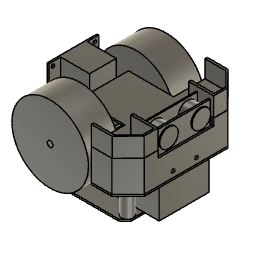
SUMO ROBOT (Autodesk Fusion 360 design; units mm, degrees)
Autodesk Fusion 360 part; units mm, degrees
note: some values were not read from the file. Chosen so that the rebuilt part matches the saved one: which face or edge a step refers to.
(part 1 of 2)
sketch "Sketch1" plane through (0, 0, 0) normal (0, 0, 1) x (1, 0, 0)
  line L0 (0, 0) -> (100, 0)
  line L1 (100, 0) -> (100, 100)
  line L2 (100, 100) -> (0, 100)
  line L3 (0, 100) -> (0, 0)
  constraint horizontal L0
  constraint vertical L1
  constraint horizontal L2
  constraint vertical L3
  constraint coincident L0.start L3.end
sketch "Sketch2" plane through (0, 0, 0) normal (0, 0, 1) x (1, 0, 0)
  line L0 (125, 0) -> (147, 0)
  line L1 (147, 0) -> (147, 19)
  line L2 (147, 19) -> (125, 19)
  line L3 (125, 19) -> (125, 0)
  dimension "d1" = 22
  dimension "d2" = 19
  constraint horizontal L0
  constraint vertical L1
  constraint horizontal L2
  constraint vertical L3
  measures "d1" distance of L0.start L0.end
  measures "d2" distance of L0.start L2.end
extrude "Extrude1" add sketch "Sketch2" against normal blind 64 makes body 1
sketch "Sketch3" plane through (0, 0, -64) normal (0, 0, -1) x (1, 0, 0)
  line L0 (125, 0) -> (125, -19)
  line L1 (125, -19) -> (147, -19)
  line L2 (147, -19) -> (147, 0)
  line L3 (147, 0) -> (125, 0)
extrude "Extrude2" cut sketch "Sketch3" against normal blind 27 bodies 1
extrude "Extrude3" add 1 faces at (132.3333, 12.6667, 0) along direction (0, 0, 1) blind 27 separate body on bodies 1 makes body 2
move_face "OffsetFaces1" offset -2.5 4 faces at (147, 6.3333, 18) (132.3333, 0, 9) (125, 12.6667, 18) (139.6667, 19, 9) on bodies 2
fillet "Fillet1" radius 5 2 edges at (147, 9.5, -37) (125, 9.5, -37) on bodies 1
sketch "Sketch4" plane through (0, 0, 0) normal (0, -1, 0) x (1, 0, 0)
  arc A0 (125, -32) -> (130, -37) centre (130, -32) ccw
  line L0 (130, -37) -> (142, -37)
  arc A1 (142, -37) -> (147, -32) centre (142, -32) ccw
  line L1 (147, -32) -> (147, 0)
  line L2 (147, 0) -> (125, 0)
  line L3 (125, 0) -> (125, -32)
  line L4 (130, -37) -> (130, -7)
  line L5 (125, -7.4905) -> (126, -7.4905)
  circle A2 centre (128, -7) radius 2
  circle A3 centre (144, -7) radius 2
  dimension "d12" = 4
  constraint coincident A0.end L0.start
  constraint perpendicular L0 L4
  constraint coincident L3 L5.start
  constraint perpendicular L3 L5
  measures "d12" diameter of A2
extrude "Extrude4" cut sketch "Sketch4" against normal blind 71 contours A2 | A3 bodies 1
sketch "Sketch5" plane through (0, 0, 0) normal (0, -1, 0) x (1, 0, 0)
  circle A0 centre (128, -7) radius 2
  circle A1 centre (144, -7) radius 2
  arc A2 (125, -32) -> (130, -37) centre (130, -32) ccw
  line L0 (130, -37) -> (142, -37)
  arc A3 (142, -37) -> (147, -32) centre (142, -32) ccw
  line L1 (147, -32) -> (147, 0)
  line L2 (147, 0) -> (125, 0)
  line L3 (125, 0) -> (125, -32)
  line L4 (136, -37) -> (136, -28)
  line L5 (136, -28) -> (136, -25.5)
  circle A4 centre (136, -25.5) radius 2.5
  dimension "d15" = 2.5
  constraint midpoint L0 L4.start
  constraint perpendicular L0 L4
  constraint parallel L4 L5
  constraint coincident L5.end A4.centre
  constraint coincident L4.end A4
  measures "d15" distance of L4.end L5.end
extrude "Extrude5" add sketch "Sketch5" along normal blind 9 and the other way blind 28 contours A4 bodies 1
sketch "Sketch6" plane through (0, -9, 0) normal (0, -1, 0) x (1, 0, 0)
  circle A0 centre (136, -25.5) radius 2.5
  circle A1 centre (136, -25.5) radius 33
  dimension "d20" = 66
  constraint concentric A0 A1
  measures "d20" diameter of A1
extrude "Extrude6" add sketch "Sketch6" along normal blind 26 separate body makes body 3
move_body "Move1" bodies 3 to x (1, 0, 0) y (0, 1, 0) z (0, 0, 1) at (0, 6, 0)
move_body "Move2" bodies 2 3 1 to x (0, 0, -1) y (0, 1, 0) z (1, 0, 0) at (135, 0, 121)
copy_body "CopyPasteBodies1" bodies 1 3 2 makes body 4 makes body 5 makes body 6
move_body "Move3" bodies 4 5 6 to x (1, 0, 0) y (0, -1, 0) z (0, 0, -1) at (0, 72, -30)
move_body "Move4" bodies 5 4 6 to x (1, 0, 0) y (0, 1, 0) z (0, 0, 1) at (-80, 0, 4)
move_body "Move5" bodies 3 1 2 to x (1, 0, 0) y (0, 1, 0) z (0, 0, 1) at (-80, 15, 4)
sketch "Sketch7" plane through (0, 0, 0) normal (0, 0, 1) x (1, 0, 0)
sketch "Sketch8" plane through (0, 0, 0) normal (0, 0, 1) x (1, 0, 0)
  line L0 (0, 72) -> (66, 72)
  line L1 (66, 72) -> (66, 15)
  line L2 (66, 15) -> (0, 15)
  line L3 (0, 15) -> (0, 72)
  line L4 (100, 100) -> (66, 100)
  line L5 (66, 100) -> (66, 0)
  line L6 (66, 0) -> (100, 0)
  line L7 (100, 0) -> (100, 100)
  constraint horizontal L0
  constraint vertical L1
  constraint horizontal L2
  constraint vertical L3
  constraint horizontal L4
  constraint vertical L5
  constraint horizontal L6
  constraint vertical L7
extrude "Extrude7" add sketch "Sketch8" along normal blind 2.5 separate body makes body 7
extrude "Extrude8" add 1 faces at (88.6667, 100, 1.6667) along direction (0, 1, 0) blind 1 on bodies 7 bodies 7
extrude "Extrude9" add 1 faces at (77.3333, 0, 1.6667) along direction (0, -1, 0) blind 14 on bodies 7 bodies 7
sketch "Sketch9" plane through (0, 53, 0) normal (0, -1, 0) x (1, 0, 0)
  circle A0 centre (29.5, -11) radius 2.5
  circle A1 centre (48, -19) radius 2
  circle A2 centre (48, -3) radius 2
  arc A3 (18, -17) -> (23, -22) centre (23, -17) ccw
  line L0 (23, -22) -> (55, -22)
  line L1 (55, -22) -> (55, 0)
  line L2 (55, 0) -> (23, 0)
  arc A4 (23, 0) -> (18, -5) centre (23, -5) ccw
  line L3 (18, -5) -> (18, -17)
  circle A5 centre (48, -19) radius 2
  circle A6 centre (48, -3) radius 2
  constraint concentric A1 A5
  constraint concentric A2 A6
sketch "Sketch10" plane through (0, 0, 0) normal (0, 0, -1) x (1, 0, 0)
  line L0 (66, 14) -> (66, -15)
  line L1 (66, -15) -> (0, -15)
  line L2 (0, -15) -> (0, -72)
  line L3 (0, -72) -> (66, -72)
  line L4 (66, -72) -> (66, -101)
  line L5 (66, -101) -> (100, -101)
  line L6 (100, -101) -> (100, 14)
  line L7 (100, 14) -> (66, 14)
  line L8 (42, -53) -> (54, -53)
  line L9 (54, -53) -> (54, -34)
  line L10 (54, -34) -> (42, -34)
  line L11 (42, -34) -> (42, -53)
  line L12 (42, -47) -> (54, -47)
  line L13 (54, -47) -> (54, -40)
  line L14 (54, -40) -> (42, -40)
  line L15 (42, -40) -> (42, -47)
  constraint horizontal L8
  constraint vertical L9
  constraint horizontal L10
  constraint vertical L11
  constraint horizontal L12
  constraint vertical L13
  constraint horizontal L14
  constraint vertical L15
  constraint coincident L9 L13.end
  constraint coincident L11 L12.start
extrude "Extrude10" add sketch "Sketch10" along normal blind 22 separate body contours L8 L9 L11 L12 | L9 L10 L11 L14 makes body 8 at (46, 47, -7.3333) makes body 9 at (50, 34, -7.3333)
extrude "Extrude11" cut sketch "Sketch9" along normal blind 40 contours A1 A5 | A2 A6 bodies 8 9
sketch "Sketch11" plane through (0, 0, 0) normal (0, 0, -1) x (1, 0, 0)
  line L0 (66, 14) -> (66, -15)
  line L1 (66, -15) -> (0, -15)
  line L2 (0, -15) -> (0, -72)
  line L3 (0, -72) -> (66, -72)
  line L4 (66, -72) -> (66, -101)
  line L5 (66, -101) -> (100, -101)
  line L6 (100, -101) -> (100, 14)
  line L7 (100, 14) -> (66, 14)
  circle A0 centre (95, -50) radius 1.5
  circle A1 centre (95, -43) radius 2
  dimension "d33" = 3
  measures "d33" diameter of A0
extrude "Extrude12" cut sketch "Sketch11" against normal blind 5 contours A0 | A1 bodies 7
sketch "Sketch12" plane through (0, 0, 0) normal (1, 0, 0) x (0, 1, 0)
  line L0 (-55, 0) -> (-100, 0)
  line L1 (-100, 0) -> (-100, 20)
  line L2 (-100, 20) -> (-55, 20)
  line L3 (-55, 20) -> (-55, 0)
  circle A0 centre (-65, 10) radius 8
  circle A1 centre (-90, 10) radius 8
  dimension "d36" = 45
  dimension "d37" = 20
  dimension "d38" = 16
  dimension "d39" = 16
  constraint horizontal L0
  constraint vertical L1
  constraint horizontal L2
  constraint vertical L3
  measures "d36" distance of L0.start L0.end
  measures "d37" distance of L0.start L2.end
  measures "d38" diameter of A0
  measures "d39" diameter of A1
extrude "Extrude13" add sketch "Sketch12" along normal blind 1 separate body makes body 10
extrude "Extrude14" add sketch "Sketch12" along normal blind 13 contours A0 | A1 bodies 10
move_body "Move6" bodies 10 to x (1, 0, 0) y (0, 1, 0) z (0, 0, 1) at (86, 121, -35)
sketch "Sketch13" plane through (87, 0, 0) normal (1, 0, 0) x (0, 1, 0)
  circle A0 centre (56, -25) radius 8
  circle A1 centre (31, -25) radius 8
  line L0 (66, -15) -> (21, -15)
  line L1 (21, -15) -> (21, -35)
  line L2 (21, -35) -> (66, -35)
  line L3 (66, -35) -> (66, -15)
  line L4 (22, -34) -> (65, -34)
  line L5 (65, -34) -> (65, 0)
  line L6 (65, 0) -> (22, 0)
  line L7 (22, 0) -> (22, -34)
  circle A2 centre (56, -25) radius 8
  circle A3 centre (31, -25) radius 8
  constraint horizontal L4
  constraint vertical L5
  constraint horizontal L6
  constraint vertical L7
  constraint concentric A0 A2
  constraint concentric A1 A3
extrude "Extrude15" add sketch "Sketch13" along normal blind 3 contours L0 L4 L5 L7 | L0 L5 L6 L7 bodies 7
chamfer "Chamfer1" distance 2 angle 45 4 edges at (90, 43.5, 0) (88.5, 65, 0) (88.5, 22, 0) (87, 43.5, 0) on bodies 7
chamfer "Chamfer2" distance 10 angle 45 2 edges at (100, -14, 1.25) (100, 101, 1.25) on bodies 7
sketch "Sketch14" plane through (0, 0, 0) normal (0, 0, -1) x (1, 0, 0)
  line L0 (90, -101) -> (100, -91)
  line L1 (100, -91) -> (100, 4)
  line L2 (100, 4) -> (90, 14)
  line L3 (90, 14) -> (66, 14)
  line L4 (66, 14) -> (66, -15)
  line L5 (66, -15) -> (0, -15)
  line L6 (0, -15) -> (0, -72)
  line L7 (0, -72) -> (66, -72)
  line L8 (66, -72) -> (66, -101)
  line L9 (66, -101) -> (90, -101)
  circle A0 centre (95, -43) radius 2
  circle A1 centre (95, -50) radius 1.5
  line L10 (85, -20) -> (92, -20)
  line L11 (92, -20) -> (92, -67)
  line L12 (92, -67) -> (85, -67)
  line L13 (85, -67) -> (85, -20)
  circle A2 centre (90, 9) radius 2
  circle A3 centre (93, 5) radius 1.5
  circle A4 centre (90, -95) radius 2
  circle A5 centre (93, -90) radius 1.5
  dimension "d48" = 3
  dimension "d49" = 3
  measures "d48" diameter of A3
  measures "d49" diameter of A5
extrude "Extrude16" cut sketch "Sketch14" against normal blind 5 contours A2 | A3 | A4 | A5 bodies 7
sketch "Sketch15" plane through (0, 0, 0) normal (1, 0, 0) x (0, 1, 0)
  line L0 (-60, 0) -> (-103, 0)
  line L1 (-103, 0) -> (-103, 43)
  line L2 (-103, 43) -> (-60, 43)
  line L3 (-60, 43) -> (-60, 0)
  line L4 (-81.5, 4.9861) -> (-70, 4.9861)
  line L5 (-70, 4.9861) -> (-70, 0)
  line L6 (-70, 0) -> (-81.5, 0)
  line L7 (-81.5, 0) -> (-81.5, 4.9861)
  line L8 (-81.5, 4.9861) -> (-93, 4.9861)
  line L9 (-93, 4.9861) -> (-93, 0)
  line L10 (-93, 0) -> (-81.5, 0)
  line L11 (-81.5, 0) -> (-81.5, 4.9861)
  line L12 (-70, 0) -> (-93, 0)
  line L13 (-93, 0) -> (-93, 16)
  line L14 (-93, 16) -> (-70, 16)
  line L15 (-70, 16) -> (-70, 0)
  dimension "d52" = 43
  dimension "d53" = 43
  constraint horizontal L0
  constraint vertical L1
  constraint horizontal L2
  constraint vertical L3
  constraint horizontal L4
  constraint vertical L5
  constraint horizontal L6
  constraint vertical L7
  constraint coincident L0 L5.end
  constraint horizontal L8
  constraint vertical L9
  constraint horizontal L10
  constraint vertical L11
  constraint coincident L0 L9.end
  constraint horizontal L12
  constraint vertical L13
  constraint horizontal L14
  constraint vertical L15
  measures "d52" distance of L0.start L0.end
  measures "d53" distance of L0.start L2.end
extrude "Extrude17" add sketch "Sketch15" along normal blind 1.5 separate body makes body 11
extrude "Extrude18" add sketch "Sketch15" against normal blind 25 contours L0 L4 L5 L6 L7 L11 L12 L15 | L0 L7 L8 L9 L10 L11 L12 L13 | L4 L8 L13 L14 L15 bodies 11
sketch "Sketch16" plane through (1.5, 0, 0) normal (1, 0, 0) x (0, 1, 0)
  line L0 (-103, 0) -> (-60, 0)
  line L1 (-60, 0) -> (-60, 43)
  line L2 (-60, 43) -> (-103, 43)
  line L3 (-103, 43) -> (-103, 0)
  line L4 (-60, 0) -> (-62, 0)
  line L5 (-60, 0) -> (-60, 2)
  line L6 (-60, 2) -> (-103, 2)
  line L7 (-62, 0) -> (-62, 43)
  circle A0 centre (-63.5, 3.5) radius 1.5
  line L8 (-101, 0) -> (-101, 43)
  line L9 (-62, 41) -> (-101, 41)
  circle A1 centre (-99.5, 3.5) radius 1.5
  circle A2 centre (-99.5, 39.5) radius 1.5
  circle A3 centre (-63.5, 39.5) radius 1.5
  constraint coincident L0.end L1.start
  constraint coincident L0 L4.end
  constraint perpendicular L1 L4
  constraint coincident L1 L5.end
  constraint coincident L3 L6.end
  constraint perpendicular L3 L6
  constraint coincident L2 L7.end
  constraint perpendicular L2 L7
  constraint tangent L6 A0
  constraint coincident L0 L8.start
  constraint coincident L2 L8.end
  constraint perpendicular L2 L8
  constraint coincident L7 L9.start
  constraint coincident L8 L9.end
  constraint perpendicular L8 L9
  constraint tangent L8 A1
  constraint tangent L8 A2
  constraint tangent L7 A3
extrude "Extrude19" cut sketch "Sketch16" against normal blind 10 contours A1 | A0 | A2 | A3 bodies 11
extrude "Extrude20" add 1 faces at (0, -85.3333, 31.2328) along direction (-1, 0, 0) blind 10 on bodies 11 bodies 11
move_body "Move7" bodies 11 to x (0, 0, -1) y (0, 1, 0) z (1, 0, 0) at (3, 125, -35)
move_body "Move8" bodies 11 to x (1, 0, 0) y (0, 1, 0) z (0, 0, 1) at (-2.5, 0, 0)
sketch "Sketch17" plane through (0, 0, -36.5) normal (0, 0, -1) x (1, 0, 0)
  circle A0 centre (4, -25.5) radius 1.5
  circle A1 centre (40, -25.5) radius 1.5
  circle A2 centre (4, -61.5) radius 1.5
  circle A3 centre (40, -61.5) radius 1.5
  line L0 (0.5, -22) -> (0.5, -65)
  line L1 (0.5, -65) -> (43.5, -65)
  line L2 (43.5, -65) -> (43.5, -22)
  line L3 (43.5, -22) -> (0.5, -22)
  circle A4 centre (4, -61.5) radius 1.5
  circle A5 centre (4, -25.5) radius 1.5
  constraint concentric A2 A4
  constraint concentric A0 A5
sketch "Sketch18" plane through (0, 0, -36.5) normal (0, 0, -1) x (1, 0, 0)
  circle A0 centre (4, -61.5) radius 3.5
  circle A1 centre (4, -25.5) radius 3.5
extrude "Extrude21" add sketch "Sketch18" against normal blind 35 separate body makes body 12 at (7.4826, 61.8485, -13.1667) makes body 13 at (7.4826, 25.8485, -13.1667)
extrude "Extrude22" cut sketch "Sketch17" against normal blind 55 contours A0 A5 | A2 A4 bodies 7 12 13
move_body "Move9" bodies 13 to x (1, 0, 0) y (0, 1, 0) z (0, 0, 1) at (0, 0, 4)
move_body "Move10" bodies 12 to x (1, 0, 0) y (0, 1, 0) z (0, 0, 1) at (0, 0, 4)
extrude "Extrude23" cut 2 faces at (3.2029, 28.2109, -32.5) (3.2029, 64.2109, -32.5) along direction (0, 0, 1) blind 10 on bodies 12 13 bodies 12 13
extrude "Extrude24" add 2 faces at (3.2029, 28.2109, -22.5) (3.2029, 64.2109, -22.5) along direction (0, 0, -1) blind 2.5 on bodies 12 13 bodies 13 12
sketch "Sketch19" plane through (0, 0, -22) normal (0, 0, -1) x (1, 0, 0)
  line L0 (42, -53) -> (54, -53)
  line L1 (54, -53) -> (54, -47)
  line L2 (54, -47) -> (42, -47)
  line L3 (42, -47) -> (42, -53)
  line L4 (42, -47) -> (54, -47)
  line L5 (54, -47) -> (54, -40)
  line L6 (54, -40) -> (42, -40)
  line L7 (42, -40) -> (42, -47)
  constraint horizontal L4
  constraint vertical L5
  constraint horizontal L6
  constraint vertical L7
  constraint coincident L2.end L3.start
extrude "Extrude25" cut sketch "Sketch19" against normal blind 37 contours L2 L4 L5 L6 L7 bodies 7
sketch "Sketch20" plane through (0, 0, 0) normal (0, 0, -1) x (1, 0, 0)
  line L0 (54, -47) -> (42, -47)
  line L1 (42, -47) -> (42, -40)
  line L2 (42, -40) -> (54, -40)
  line L3 (54, -40) -> (54, -47)
  circle A0 centre (4, -61.5) radius 1.5
  circle A1 centre (4, -25.5) radius 1.5
  circle A2 centre (93, 5) radius 1.5
  circle A3 centre (90, -95) radius 2
  circle A4 centre (90, 9) radius 2
  circle A5 centre (93, -90) radius 1.5
  line L4 (90, -101) -> (100, -91)
  line L5 (100, -91) -> (100, 4)
  line L6 (100, 4) -> (90, 14)
  line L7 (90, 14) -> (66, 14)
  line L8 (66, 14) -> (66, -15)
  line L9 (66, -15) -> (0, -15)
  line L10 (0, -15) -> (0, -72)
  line L11 (0, -72) -> (66, -72)
  line L12 (66, -72) -> (66, -101)
  line L13 (66, -101) -> (90, -101)
  circle A6 centre (95, -43) radius 2
  circle A7 centre (95, -50) radius 1.5
  line L14 (85, -20) -> (92, -20)
  line L15 (92, -20) -> (92, -67)
  line L16 (92, -67) -> (85, -67)
  line L17 (85, -67) -> (85, -20)
  circle A8 centre (75.2156, -86.5) radius 5
  circle A9 centre (75.2156, -0.5) radius 5
  dimension "d72" = 10
  dimension "d73" = 10
  measures "d72" diameter of A8
  measures "d73" diameter of A9
extrude "Extrude26" add sketch "Sketch20" along normal blind 40 contours A8 | A9 bodies 7
extrude "Extrude27" add 2 faces at (3.2029, 28.2109, -25) (3.2029, 64.2109, -25) along direction (0, 0, -1) blind 10 on bodies 12 13 bodies 13 12
sketch "Sketch21" plane through (0, 0, -40) normal (0, 0, -1) x (1, 0, 0)
  circle A0 centre (75.2156, -86.5) radius 5
  circle A1 centre (75.2156, -86.5) radius 1.5
  dimension "d78" = 3
  constraint concentric A0 A1
  measures "d78" diameter of A1
sketch "Sketch22" plane through (0, 0, -40) normal (0, 0, -1) x (1, 0, 0)
  circle A0 centre (75.2156, -0.5) radius 5
  circle A1 centre (75.2156, -0.5) radius 1.5
  dimension "d79" = 3
  constraint concentric A0 A1
  measures "d79" diameter of A1
extrude "Extrude28" cut sketch "Sketch22" sketch "Sketch21" against normal blind 72 contours A1 of sketch 2 contours A1 bodies 7
sketch "Sketch23" plane through (0, 0, -40) normal (0, 0, -1) x (1, 0, 0)
  circle A0 centre (75.2156, -86.5) radius 1.5
  circle A1 centre (75.2156, -86.5) radius 5
  line L0 (65, -101) -> (65, -72)
  line L1 (65, -72) -> (0, -72)
  line L2 (0, -72) -> (0, -15)
  line L3 (0, -15) -> (66, -15)
  line L4 (66, -15) -> (65, -15)
  line L5 (65, -15) -> (65, 14)
  line L6 (65, 14) -> (90, 14)
  line L7 (90, 14) -> (100, 4)
  line L8 (100, 4) -> (100, -91)
  line L9 (100, -91) -> (90, -101)
  line L10 (90, -101) -> (65, -101)
  constraint vertical L0
  constraint perpendicular L0 L1
  constraint perpendicular L1 L2
  constraint perpendicular L2 L3
  constraint coincident L3 L4.end
  constraint perpendicular L3 L5
  constraint perpendicular L5 L6
  constraint perpendicular L6 L8
  constraint perpendicular L7 L9
  constraint perpendicular L0 L10
extrude "Extrude29" add sketch "Sketch23" along normal blind 2.5 contours A1 | L0 L1 L2 L3 L5 L6 L7 L8 L9 L10 bodies 7
extrude "Extrude30" cut sketch "Sketch22" along normal blind 4 contours A1 bodies 7
sketch "Sketch24" plane through (0, 0, 0) normal (0, 0, 1) x (1, 0, 0)
  line L0 (-50, 0) -> (-115, 0)
  line L1 (-115, 0) -> (-115, 55)
  line L2 (-115, 55) -> (-50, 55)
  line L3 (-50, 55) -> (-50, 0)
  dimension "d86" = 65
  dimension "d87" = 55
  constraint horizontal L0
  constraint vertical L1
  constraint horizontal L2
  constraint vertical L3
  measures "d86" distance of L0.start L0.end
  measures "d87" distance of L0.start L2.end
sketch "Sketch25" plane through (0, 0, 0) normal (0, 0, 1) x (1, 0, 0)
extrude "Extrude31" add sketch "Sketch24" against normal blind 20 separate body makes body 14
chamfer "Chamfer3" distance 5 angle 45 4 edges at (-82.5, 0, -20) (-82.5, 55, -20) (-82.5, 0, 0) (-82.5, 55, 0) on bodies 14
move_body "Move11" bodies 14 to x (1, 0, 0) y (0, 1, 0) z (0, 0, 1) at (115, 17.5, -45)
sketch "Sketch26" plane through (0, 0, 0) normal (0, 1, 0) x (1, 0, 0)
  line L0 (-50, 0) -> (-117, 0)
  line L1 (-117, 0) -> (-117, -54)
  line L2 (-117, -54) -> (-50, -54)
  line L3 (-50, -54) -> (-50, 0)
  dimension "d91" = 67
  dimension "d92" = 54
  constraint horizontal L0
  constraint vertical L1
  constraint horizontal L2
  constraint vertical L3
  measures "d91" distance of L0.start L0.end
  measures "d92" distance of L0.start L2.end
extrude "Extrude32" add sketch "Sketch26" along normal blind 10 separate body makes body 15
move_body "Move12" bodies 15 to x (1, 0, 0) y (0, 0, 1) z (0, -1, 0) at (120, 72, -75)
sketch "Sketch27" plane through (0, 0, -75) normal (0, 0, -1) x (1, 0, 0)
  line L0 (70, -72) -> (70, -18)
  line L1 (70, -18) -> (3, -18)
  line L2 (3, -18) -> (3, -72)
  line L3 (3, -72) -> (70, -72)
  line L4 (3, -64.7927) -> (70, -64.7927)
  line L5 (70, -64.7927) -> (70, -25)
  line L6 (70, -25) -> (3, -25)
  line L7 (3, -25) -> (3, -64.7927)
  constraint horizontal L4
  constraint vertical L5
  constraint horizontal L6
  constraint vertical L7
  constraint coincident L0 L5.end
  constraint coincident L2 L4.start
extrude "Extrude33" cut sketch "Sketch27" against normal blind 5 contours L0 L2 L4 L5 L6 L7 bodies 15
move_body "Move13" bodies 14 15 to x (1, 0, 0) y (0, 1, 0) z (0, 0, 1) at (0, 0, 3)
sketch "Sketch28" plane through (100, 0, 0) normal (1, 0, 0) x (0, 1, 0)
  line L0 (91, -40) -> (-4, -40)
  line L1 (-4, -40) -> (-4, -42.5)
  line L2 (-4, -42.5) -> (91, -42.5)
  line L3 (91, -42.5) -> (91, -40)
  line L4 (-15.0228, -40) -> (107, -40)
  line L5 (107, -40) -> (107, -39.8)
  line L6 (107, -39.8) -> (-15.0228, -39.8)
  line L7 (-15.0228, -39.8) -> (-15.0228, -40)
  dimension "d97" = 0.2
  constraint horizontal L4
  constraint vertical L5
  constraint horizontal L6
  constraint vertical L7
  measures "d97" distance of L4.start L6.end
extrude "Extrude34" cut sketch "Sketch28" against normal blind 113 contours L0 L4 L5 L6 L7 bodies 7 makes body 16 at (17.3556, 42.3333, 2.5)
move_face "OffsetFaces2" offset -0.3 2 faces at (88, 63.9602, -25.7965) (89, 35.6699, -18.5045) on bodies 16
sketch "Sketch29" plane through (0, 53, 0) normal (0, 1, 0) x (-1, 0, 0)
  circle A0 centre (-48, -19) radius 2
  circle A1 centre (-48, -3) radius 2
  line L0 (-42, 0) -> (-54, 0)
  line L1 (-54, 0) -> (-54, -22)
  line L2 (-54, -22) -> (-42, -22)
  line L3 (-42, -22) -> (-42, 0)
  line L4 (-42, -22) -> (-42, 0)
  line L5 (-35, 0) -> (-42, -22)
  line L6 (-54, -22) -> (-54, 0)
  line L7 (-60, 0) -> (-54, -22)
  line L8 (-54, 0) -> (-60, 0)
  line L9 (-35, 0) -> (-42, 0)
  constraint coincident L2.end L3.start
  constraint coincident L0.start L3.end
  constraint coincident L1.end L2.start
  constraint coincident L0.end L1.start
  constraint perpendicular L6 L8
  constraint perpendicular L4 L9
extrude "Extrude35" add sketch "Sketch29" against normal blind 19 contours L3 L4 L5 L9 | L1 L6 L7 L8 bodies 8 9 16
sketch "Sketch30" plane through (0, 0, -22) normal (0, 0, -1) x (1, 0, 0)
  line L0 (42, -53) -> (54, -53)
  line L1 (54, -53) -> (54, -47)
  line L2 (54, -47) -> (42, -47)
  line L3 (42, -47) -> (42, -53)
  line L4 (65, -40) -> (30, -40)
  line L5 (30, -40) -> (30, -47)
  line L6 (30, -47) -> (65, -47)
  line L7 (65, -47) -> (65, -40)
  constraint horizontal L4
  constraint vertical L5
  constraint horizontal L6
  constraint vertical L7
extrude "Extrude36" cut sketch "Sketch30" against normal blind 34 contours L2 L4 L5 L6 L7 bodies 8
sketch "Sketch31" plane through (0, 0, 2.5) normal (0, 0, 1) x (-1, 0, 0)
  line L0 (-65, -40) -> (-30, -40)
  line L1 (-30, -40) -> (-30, -47)
  line L2 (-30, -47) -> (-65, -47)
  line L3 (-65, -47) -> (-65, -40)
  circle A0 centre (-75.2156, -0.5) radius 1.5
  circle A1 centre (-75.2156, -86.5) radius 1.5
  circle A2 centre (-4, -61.5) radius 1.5
  circle A3 centre (-4, -25.5) radius 1.5
  circle A4 centre (-93, 5) radius 1.5
  circle A5 centre (-90, -95) radius 2
  circle A6 centre (-90, 9) radius 2
  circle A7 centre (-93, -90) radius 1.5
  line L4 (-100, -91) -> (-90, -101)
  line L5 (-90, -101) -> (-66, -101)
  line L6 (-66, -101) -> (-66, -72)
  line L7 (-66, -72) -> (0, -72)
  line L8 (0, -72) -> (0, -15)
  line L9 (0, -15) -> (-66, -15)
  line L10 (-66, -15) -> (-66, 14)
  line L11 (-66, 14) -> (-90, 14)
  line L12 (-90, 14) -> (-100, 4)
  line L13 (-100, 4) -> (-100, -91)
  circle A8 centre (-95, -50) radius 1.5
  circle A9 centre (-95, -43) radius 2
  line L14 (-90, -55) -> (-80, -55)
  line L15 (-80, -55) -> (-80, -31)
  line L16 (-80, -31) -> (-90, -31)
  line L17 (-90, -31) -> (-90, -55)
  line L18 (-90, -55) -> (-80, -55)
  line L19 (-80, -55) -> (-80, -52)
  line L20 (-80, -52) -> (-90, -52)
  line L21 (-90, -52) -> (-90, -55)
  line L22 (-90, -31) -> (-80, -31)
  line L23 (-80, -31) -> (-80, -34)
  line L24 (-80, -34) -> (-90, -34)
  line L25 (-90, -34) -> (-90, -31)
  constraint horizontal L14
  constraint vertical L15
  constraint horizontal L16
  constraint vertical L17
  constraint horizontal L18
  constraint vertical L19
  constraint horizontal L20
  constraint vertical L21
  constraint coincident L15 L19.end
  constraint horizontal L22
  constraint vertical L23
  constraint horizontal L24
  constraint vertical L25
  constraint coincident L15 L23.end
extrude "Extrude37" add sketch "Sketch31" along normal blind 17 separate body contours L14 L15 L17 L18 L19 L20 L21 | L15 L16 L17 L22 L23 L24 L25 makes body 17 at (83.3333, 52, 8.1667) makes body 18 at (83.3333, 31, 8.1667)
sketch "Sketch32" plane through (0, 31, 0) normal (0, -1, 0) x (1, 0, 0)
  line L0 (80, 2.5) -> (90, 2.5)
  line L1 (90, 2.5) -> (90, 19.5)
  line L2 (90, 19.5) -> (80, 19.5)
  line L3 (80, 19.5) -> (80, 2.5)
  circle A0 centre (85, 15) radius 1.5
  dimension "d107" = 3
  measures "d107" diameter of A0
extrude "Extrude38" cut sketch "Sketch32" against normal blind 49 contours A0 bodies 17 18
chamfer "Chamfer4" distance 2 angle 45 4 edges at (80, 53.5, 19.5) (90, 53.5, 19.5) (90, 32.5, 19.5) (80, 32.5, 19.5) on bodies 17 18
sketch "Sketch33" plane through (0, 55, 0) normal (0, 1, 0) x (-1, 0, 0)
  line L0 (-88, 19.5) -> (-90, 17.5)
  line L1 (-90, 17.5) -> (-90, 2.5)
  line L2 (-90, 2.5) -> (-80, 2.5)
  line L3 (-80, 2.5) -> (-80, 17.5)
  line L4 (-80, 17.5) -> (-82, 19.5)
  line L5 (-82, 19.5) -> (-88, 19.5)
  circle A0 centre (-85, 15) radius 1.5
sketch "Sketch34" plane through (0, 0, 0) normal (1, 0, 0) x (0, 1, 0)
  line L0 (-50, -20) -> (-62, -20)
  line L1 (-62, -20) -> (-62, -3)
  line L2 (-62, -3) -> (-50, -3)
  line L3 (-50, -3) -> (-50, -20)
  line L4 (-56, -20) -> (-50, -13)
  line L5 (-56, -3) -> (-50, -10)
  line L6 (-56, -20) -> (-62, -13)
  line L7 (-62, -10) -> (-56, -3)
  line L8 (-56, -20) -> (-57.5, -20)
  line L9 (-57.5, -20) -> (-57.5, -3)
  line L10 (-57.5, -3) -> (-56, -3)
  line L11 (-56, -3) -> (-56, -20)
  line L12 (-56, -20) -> (-54.5, -20)
  line L13 (-54.5, -20) -> (-54.5, -3)
  line L14 (-54.5, -3) -> (-56, -3)
  line L15 (-56, -3) -> (-56, -20)
  dimension "d111" = 1.5
  dimension "d112" = 1.5
  constraint horizontal L0
  constraint vertical L1
  constraint horizontal L2
  constraint vertical L3
  constraint midpoint L0 L4.start
  constraint coincident L3 L4.end
  constraint midpoint L2 L5.start
  constraint coincident L3 L5.end
  constraint coincident L1 L6.end
  constraint parallel L5 L6
  constraint parallel L4 L7
  constraint horizontal L8
  constraint vertical L9
  constraint horizontal L10
  constraint vertical L11
  constraint horizontal L12
  constraint vertical L13
  constraint horizontal L14
  constraint vertical L15
  measures "d111" distance of L4.start L8.end
  measures "d112" distance of L4.start L12.end
revolve "Revolve1" add sketch "Sketch34" angle 360 about axis through (0, -56, -3) along (0, 0, -1) separate body contours L3 L4 L5 L13 makes body 19
move_body "Move14" bodies 19 to x (1, 0, 0) y (0, 0, -1) z (0, 1, 0) at (85, 56.25, -40.95)
move_body "Move15" bodies 19 to x (1, 0, 0) y (0, 1, 0) z (0, 0, 1) at (0, -1.5, 0)
sketch "Sketch35" plane through (0, -14, 0) normal (0, -1, 0) x (1, 0, 0)
  circle A0 centre (29.5, -11) radius 2.5
  circle A1 centre (29.5, -11) radius 33
sketch "Sketch36" plane through (0, 0, 2.5) normal (0, 0, 1) x (-1, 0, 0)
  line L0 (-65, -40) -> (-30, -40)
  line L1 (-30, -40) -> (-30, -47)
  line L2 (-30, -47) -> (-65, -47)
  line L3 (-65, -47) -> (-65, -40)
  circle A0 centre (-75.2156, -0.5) radius 1.5
  circle A1 centre (-75.2156, -86.5) radius 1.5
  circle A2 centre (-4, -61.5) radius 1.5
  circle A3 centre (-4, -25.5) radius 1.5
  circle A4 centre (-93, 5) radius 1.5
  circle A5 centre (-90, -95) radius 2
  circle A6 centre (-90, 9) radius 2
  circle A7 centre (-93, -90) radius 1.5
  line L4 (-100, -91) -> (-90, -101)
  line L5 (-90, -101) -> (-66, -101)
  line L6 (-66, -101) -> (-66, -72)
  line L7 (-66, -72) -> (0, -72)
  line L8 (0, -72) -> (0, -15)
  line L9 (0, -15) -> (-66, -15)
  line L10 (-66, -15) -> (-66, 14)
  line L11 (-66, 14) -> (-90, 14)
  line L12 (-90, 14) -> (-100, 4)
  line L13 (-100, 4) -> (-100, -91)
  circle A8 centre (-95, -50) radius 1.5
  circle A9 centre (-95, -43) radius 2
  line L14 (-66, -101) -> (-66, -102.5)
  line L15 (-66, -102.5) -> (-90, -102.5)
  line L16 (-90, -102.5) -> (-101.5, -91)
  line L17 (-101.5, -91) -> (-101.5, 4)
  line L18 (-101.5, 4) -> (-90, 15.5)
  line L19 (-90, 15.5) -> (-66, 15.5)
  line L20 (-66, 15.5) -> (-66, 14)
  constraint coincident L5.end L6.start
  constraint perpendicular L5 L14
  constraint perpendicular L6 L15
  constraint perpendicular L15 L17
  constraint parallel L12 L18
  constraint perpendicular L17 L19
  constraint coincident L10.end L11.start
  constraint perpendicular L11 L20
extrude "Extrude39" add sketch "Sketch36" against normal blind 15 separate body contours L4 L5 L11 L12 L13 L14 L15 L16 L17 L18 L19 L20 makes body 20
sketch "Sketch37" plane through (0, 102.5, 0) normal (0, 1, 0) x (-1, 0, 0)
  line L0 (-66, 2.5) -> (-90, 2.5)
  line L1 (-90, 2.5) -> (-90, -12.5)
  line L2 (-90, -12.5) -> (-66, -12.5)
  line L3 (-66, -12.5) -> (-66, 2.5)
  line L4 (-101.5, 2.5) -> (-120, 20)
  line L5 (-120, 20) -> (-118, 20)
  line L6 (-118, 20) -> (-100, 2.5)
  line L7 (-100, 2.5) -> (-101.5, 2.5)
  constraint horizontal L5
  constraint parallel L5 L7
extrude "Extrude40" add sketch "Sketch37" against normal blind 106.5 contours L4 L5 L6 L7 bodies 20
extrude "Extrude41" cut 1 faces at (113.1667, 102.5, 14.1667) along direction (0, -1, 0) blind 11.5 on bodies 20 bodies 20
sketch "Sketch38" plane through (0, 102.5, 0) normal (0, 1, 0) x (-1, 0, 0)
  line L0 (-66, 2.5) -> (-90, 2.5)
  line L1 (-90, 2.5) -> (-90, -12.5)
  line L2 (-90, -12.5) -> (-66, -12.5)
  line L3 (-66, -12.5) -> (-66, 2.5)
  line L4 (-90, 2.5) -> (-108.5, 20)
  line L5 (-108.5, 20) -> (-106.5, 20)
  line L6 (-106.5, 20) -> (-88.5, 2.5)
  constraint coincident L0.end L1.start
  constraint perpendicular L1 L5
  constraint coincident L0 L6.end
loft "Loft1" add profiles "Sketch38" section 1 face at (113.1667, 91, 14.1667) section 2 contours L0 L4 L5 L6 on bodies 20 bodies 20
sketch "Sketch39" plane through (0, -15.5, 0) normal (0, -1, 0) x (1, 0, 0)
  line L0 (90, 2.5) -> (66, 2.5)
  line L1 (66, 2.5) -> (66, -12.5)
  line L2 (66, -12.5) -> (90, -12.5)
  line L3 (90, -12.5) -> (90, 2.5)
  line L4 (90, 2.5) -> (108.5, 20)
  line L5 (108.5, 20) -> (106.5, 20)
  line L6 (106.5, 20) -> (88.5, 2.5)
  constraint coincident L0.start L3.end
  constraint perpendicular L3 L5
  constraint coincident L0 L6.end
loft "Loft2" add profiles "Sketch39" section 1 face at (113.1667, -4, 14.1667) section 2 contours L0 L4 L5 L6 on bodies 20 bodies 20
sketch "Sketch40" plane through (0, 102.5, 0) normal (0, 1, 0) x (-1, 0, 0)
  line L0 (-66, 2.5) -> (-88.5, 2.5)
  line L1 (-88.5, 2.5) -> (-106.5, 20)
  line L2 (-106.5, 20) -> (-108.5, 20)
  line L3 (-108.5, 20) -> (-90, 2.5)
  line L4 (-90, 2.5) -> (-90, -12.5)
  line L5 (-90, -12.5) -> (-66, -12.5)
  line L6 (-66, -12.5) -> (-66, 2.5)
  line L7 (-66, 2.5) -> (-88.5, 2.5)
  line L8 (-88.5, 2.5) -> (-106.5, 20)
  line L9 (-106.5, 20) -> (-66, 20)
  line L10 (-66, 20) -> (-55, 20)
  line L11 (-55, 20) -> (-66, 2.5)
  constraint coincident L0.start L6.end
  constraint coincident L0.end L1.start
  constraint coincident L1.end L2.start
  constraint parallel L2 L9
  constraint perpendicular L6 L10
extrude "Extrude42" add sketch "Sketch40" against normal blind 1.5 separate body contours L0 L1 L7 L8 L9 L10 L11 makes body 21
sketch "Sketch41" plane through (0, -15.5, 0) normal (0, -1, 0) x (1, 0, 0)
  line L0 (88.5, 2.5) -> (66, 2.5)
  line L1 (66, 2.5) -> (66, -12.5)
  line L2 (66, -12.5) -> (90, -12.5)
  line L3 (90, -12.5) -> (90, 2.5)
  line L4 (90, 2.5) -> (108.5, 20)
  line L5 (108.5, 20) -> (106.5, 20)
  line L6 (106.5, 20) -> (88.5, 2.5)
  line L7 (66, 2.5) -> (55, 20)
  line L8 (55, 20) -> (106.5, 20)
  line L9 (66, 2.5) -> (88.5, 2.5)
  line L10 (106.5, 20) -> (88.5, 2.5)
  constraint coincident L0.end L1.start
  constraint coincident L5.end L6.start
  constraint parallel L5 L8
  constraint coincident L0.start L6.end
extrude "Extrude43" add sketch "Sketch41" against normal blind 1.5 separate body contours L0 L6 L7 L8 L9 L10 makes body 22
sketch "Sketch42" plane through (0, 0, 20) normal (0, 0, 1) x (-1, 0, 0)
  line L0 (-106.5, -102.5) -> (-55, -102.5)
  line L1 (-55, -102.5) -> (-55, -101)
  line L2 (-55, -101) -> (-106.5, -101)
  line L3 (-106.5, -101) -> (-106.5, -102.5)
  line L4 (-108, -101) -> (-106.5, -101)
  line L5 (-106.5, -102.5) -> (-108, -101)
  constraint coincident L2.end L3.start
  constraint coincident L0.start L3.end
loft "Loft3" add profiles "Sketch42" section 1 contours L3 L4 L5 section 2 face at (81.5, 101.5, 2.5) on bodies 20 bodies 20 21
sketch "Sketch43" plane through (0, 0, 20) normal (0, 0, 1) x (-1, 0, 0)
  line L0 (-55, 15.5) -> (-106.5, 15.5)
  line L1 (-106.5, 15.5) -> (-106.5, 14)
  line L2 (-106.5, 14) -> (-55, 14)
  line L3 (-55, 14) -> (-55, 15.5)
  line L4 (-106.5, 15.5) -> (-106.5, 14)
  line L5 (-106.5, 14) -> (-108, 14)
  line L6 (-108, 14) -> (-106.5, 15.5)
  constraint coincident L0.end L1.start
  constraint coincident L1.end L2.start
  constraint perpendicular L1 L5
sketch "Sketch44" plane through (0, 0, 2.5) normal (0, 0, 1) x (-1, 0, 0)
  line L0 (-88.5, 15.5) -> (-90, 14)
  line L1 (-90, 14) -> (-66, 14)
  line L2 (-66, 14) -> (-66, 15.5)
  line L3 (-66, 15.5) -> (-88.5, 15.5)
  line L4 (-90, 14) -> (-88.5, 15.5)
  line L5 (-88.5, 14) -> (-90, 14)
  line L6 (-88.5, 14) -> (-88.5, 15.5)
  constraint coincident L0.end L1.start
  constraint coincident L0.start L3.end
  constraint coincident L1 L5.start
  constraint parallel L1 L5
  constraint perpendicular L3 L6
loft "Loft4" add profiles "Sketch44", "Sketch43" section 1 contours L0 L1 L4 L5 L6 section 2 contours L1 L4 L5 L6 bodies 22 20
extrude "Extrude44" cut 1 faces at (28.4906, 44, -10.176) along direction (0, 1, 0) blind 10 on bodies 4 bodies 4
extrude "Extrude45" cut 1 faces at (28.4906, 43, -11.824) along direction (0, -1, 0) blind 10 on bodies 1 bodies 1
move_body "Move16" bodies 6 4 5 to x (1, 0, 0) y (0, 1, 0) z (0, 0, 1) at (0, -15, 0)
move_body "Move17" bodies 11 to x (1, 0, 0) y (0, 1, 0) z (0, 0, 1) at (-65, 0, 0)
extrude "Extrude46" cut 1 faces at (-33.2672, 47.3333, -25) along direction (0, 0, -1) blind 10 on bodies 11 bodies 11
move_body "Move18" bodies 11 to x (1, 0, 0) y (0, 1, 0) z (0, 0, 1) at (30, -7.5, 30)
move_body "Move19" bodies 11 to x (0, 0, -1) y (0, 1, 0) z (1, 0, 0) at (7, 0, -17.5)
move_body "Move20" bodies 10 to x (1, 0, 0) y (0, 1, 0) z (0, 0, 1) at (0, -7.5, 25)
sketch "Sketch45" plane through (0, 0, -22) normal (0, 0, -1) x (1, 0, 0)
  line L0 (23, -15) -> (23, -34)
  line L1 (23, -34) -> (55, -34)
  line L2 (55, -34) -> (55, -15)
  line L3 (55, -15) -> (23, -15)
sketch "Sketch46" plane through (0, 0, -22) normal (0, 0, -1) x (1, 0, 0)
  line L0 (23, -15) -> (23, -34)
  line L1 (23, -34) -> (55, -34)
  line L2 (55, -34) -> (55, -15)
  line L3 (55, -15) -> (23, -15)
  line L4 (150, 20) -> (225, 20)
  line L5 (225, 20) -> (225, -23)
  line L6 (225, -23) -> (150, -23)
  line L7 (150, -23) -> (150, 20)
  dimension "d130" = 75
  dimension "d131" = 43
  constraint horizontal L4
  constraint vertical L5
  constraint horizontal L6
  constraint vertical L7
  measures "d130" distance of L4.start L4.end
  measures "d131" distance of L4.start L6.end
extrude "Extrude47" add sketch "Sketch46" along normal blind 26 separate body contours L4 L5 L6 L7 makes body 23
sketch "Sketch47" plane through (0, 0, -22) normal (0, 0, -1) x (1, 0, 0)
  line L0 (5, -15) -> (85, -15)
  line L1 (85, -15) -> (85, -57)
  line L2 (85, -57) -> (5, -57)
  line L3 (5, -57) -> (5, -15)
  dimension "d134" = 80
  dimension "d135" = 42
  constraint horizontal L0
  constraint vertical L1
  constraint horizontal L2
  constraint vertical L3
  measures "d134" distance of L0.start L0.end
  measures "d135" distance of L0.start L2.end
extrude "Extrude48" add sketch "Sketch47" along normal blind 1.5 separate body makes body 24
sketch "Sketch48" plane through (5, 0, 0) normal (-1, 0, 0) x (0, -1, 0)
  line L0 (-15, -22) -> (-57, -22)
  line L1 (-57, -22) -> (-57, -23.5)
  line L2 (-57, -23.5) -> (-15, -23.5)
  line L3 (-15, -23.5) -> (-15, -22)
  line L4 (-15, -27) -> (-57, -27)
  line L5 (-57, -27) -> (-57, -17)
  line L6 (-57, -17) -> (-15, -17)
  line L7 (-15, -17) -> (-15, -27)
  constraint horizontal L4
  constraint vertical L5
  constraint horizontal L6
  constraint vertical L7
extrude "Extrude49" add sketch "Sketch48" against normal blind 7 contours L0 L5 L6 L7 | L2 L4 L5 L7 bodies 24
move_body "Move21" bodies 11 to x (1, 0, 0) y (0, 1, 0) z (0, 0, 1) at (0, 0, 3)
extrude "Extrude50" cut 1 faces at (7.3333, 29, -27) along direction (0, 0, 1) blind 3.5 on bodies 24 bodies 24
sketch "Sketch49" plane through (0.5, 0, 0) normal (-1, 0, 0) x (0, -1, 0)
  circle A0 centre (-18, 16.5) radius 1.5
  circle A1 centre (-18, -19.5) radius 1.5
  circle A2 centre (-54, 16.5) radius 1.5
  circle A3 centre (-54, -19.5) radius 1.5
  line L0 (-14.5, 20) -> (-57.5, 20)
  line L1 (-57.5, 20) -> (-57.5, -23)
  line L2 (-57.5, -23) -> (-14.5, -23)
  line L3 (-14.5, -23) -> (-14.5, 20)
  circle A4 centre (-18, -19.5) radius 1.5
  circle A5 centre (-54, -19.5) radius 1.5
  constraint concentric A1 A4
  constraint concentric A3 A5
extrude "Extrude51" cut sketch "Sketch49" against normal blind 13 contours A1 A4 | A3 A5 bodies 24
move_body "Move22" bodies 11 to x (1, 0, 0) y (0, 1, 0) z (0, 0, 1) at (-2, 0, 0)
extrude "Extrude52" add 1 faces at (5, 41.75, -22.5997) along direction (-1, 0, 0) blind 4 on bodies 24 bodies 24
sketch "Sketch50" plane through (0, 0, -23.5) normal (0, 0, -1) x (1, 0, 0)
  line L0 (1, -57) -> (85, -57)
  line L1 (85, -57) -> (85, -15)
  line L2 (85, -15) -> (1, -15)
  line L3 (1, -15) -> (1, -57)
move_body "Move23" bodies 23 to x (1, 0, 0) y (0, 1, 0) z (0, 0, 1) at (-150, 34.5, 0)
move_body "Move24" bodies 23 to x (1, 0, 0) y (0, 1, 0) z (0, 0, 1) at (0, 0, -2)
sketch "Sketch51" plane through (0, 0, -23.5) normal (0, 0, -1) x (1, 0, 0)
  line L0 (-3.3501, 13.9831) -> (96.6499, 13.9831)
  line L1 (96.6499, 13.9831) -> (96.6499, -86.0837)
  line L2 (96.6499, -86.0837) -> (-3.3501, -86.0837)
  line L3 (-3.3501, -86.0837) -> (-3.3501, 13.9831)
  line L4 (65, -15) -> (65, 13.9831)
  line L5 (65, -15) -> (85, -15)
  line L6 (85, -15) -> (85, -57)
  line L7 (85, -57) -> (65, -57)
  line L8 (65, -57) -> (65, -86.0837)
  dimension "d146" = 100
  constraint horizontal L0
  constraint vertical L1
  constraint horizontal L2
  constraint vertical L3
  constraint coincident L0 L4.end
  constraint perpendicular L0 L4
  constraint perpendicular L4 L5
  constraint perpendicular L5 L6
  constraint perpendicular L6 L7
  constraint coincident L2 L8.end
  constraint perpendicular L2 L8
  measures "d146" distance of L0.start L0.end
extrude "Extrude53" add sketch "Sketch51" against normal blind 1.5 contours L0 L1 L2 L4 L5 L6 L7 L8 bodies 24
sketch "Sketch52" plane through (0, 58.5, 0) normal (0, 1, 0) x (-1, 0, 0)
  line L0 (-86, -10) -> (-86, 10)
  line L1 (-86, 10) -> (-87, 10)
  line L2 (-87, 10) -> (-87, -10)
  line L3 (-87, -10) -> (-86, -10)
  line L4 (-87, -10) -> (-81, -10)
  line L5 (-81, -10) -> (-81, 10)
  line L6 (-81, 10) -> (-87, 10)
  line L7 (-87, 10) -> (-87, -10)
  constraint horizontal L4
  constraint vertical L5
  constraint horizontal L6
  constraint vertical L7
  constraint coincident L2.end L3.start
move_body "Move25" bodies 10 to x (1, 0, 0) y (0, 1, 0) z (0, 0, 1) at (-3, 0, 9)
chamfer "Chamfer5" distance 14 angle 45 2 edges at (96.6499, 86.0837, -22.75) (96.6499, -13.9831, -22.75) on bodies 24
sketch "Sketch53" plane through (0, 0, -22) normal (0, 0, 1) x (-1, 0, 0)
  line L0 (-82.6499, 13.9831) -> (-96.6499, -0.0169)
  line L1 (-96.6499, -0.0169) -> (-96.6499, -72.0837)
  line L2 (-96.6499, -72.0837) -> (-82.6499, -86.0837)
  line L3 (-82.6499, -86.0837) -> (-65, -86.0837)
  line L4 (-65, -86.0837) -> (-65, -57)
  line L5 (-65, -57) -> (-12, -57)
  line L6 (-12, -57) -> (-12, -15)
  line L7 (-12, -15) -> (-65, -15)
  line L8 (-65, -15) -> (-65, 13.9831)
  line L9 (-65, 13.9831) -> (-82.6499, 13.9831)
  circle A0 centre (-84.7976, -71.5419) radius 5
  circle A1 centre (-84.957, -0.5084) radius 5
  dimension "d150" = 10
  dimension "d151" = 10
  measures "d150" diameter of A0
  measures "d151" diameter of A1
extrude "Extrude54" add sketch "Sketch53" along normal blind 30 contours A0 | A1 bodies 24
sketch "Sketch54" plane through (1, 0, 0) normal (-1, 0, 0) x (0, -1, 0)
  circle A0 centre (-18, -19.5) radius 1.5
  circle A1 centre (-54, -19.5) radius 1.5
  line L0 (-57, -23.5) -> (-15, -23.5)
  line L1 (-15, -23.5) -> (-15, -17)
  line L2 (-15, -17) -> (-57, -17)
  line L3 (-57, -17) -> (-57, -23.5)
  line L4 (-20.0531, -23.5) -> (-52, -23.5)
  line L5 (-52, -23.5) -> (-52, -17)
  line L6 (-52, -17) -> (-20.0531, -17)
  line L7 (-20.0531, -17) -> (-20.0531, -23.5)
  constraint horizontal L4
  constraint vertical L5
  constraint horizontal L6
  constraint vertical L7
  constraint coincident L2 L5.end
  constraint coincident L0 L4.start
extrude "Extrude55" cut sketch "Sketch54" against normal blind 17 contours L0 L2 L4 L5 L6 L7 bodies 24
chamfer "Chamfer6" distance 3 angle 45 1 edges at (12, 54.5, -22) on bodies 24
chamfer "Chamfer7" distance 3 angle 45 1 edges at (12, 17.5266, -22) on bodies 24
extrude "Extrude56" cut 2 faces at (83.476, 70.8459, 8) (86.3676, 0.9997, 8) along direction (0, 0, -1) blind 30 on bodies 24 bodies 24
sketch "Sketch55" plane through (0, 0, -22) normal (0, 0, 1) x (-1, 0, 0)
  line L0 (-15, -20.0531) -> (-15, -15)
  line L1 (-15, -15) -> (-65, -15)
  line L2 (-65, -15) -> (-65, 13.9831)
  line L3 (-65, 13.9831) -> (-82.6499, 13.9831)
  line L4 (-82.6499, 13.9831) -> (-96.6499, -0.0169)
  line L5 (-96.6499, -0.0169) -> (-96.6499, -72.0837)
  line L6 (-96.6499, -72.0837) -> (-82.6499, -86.0837)
  line L7 (-82.6499, -86.0837) -> (-65, -86.0837)
  line L8 (-65, -86.0837) -> (-65, -57)
  line L9 (-65, -57) -> (-15, -57)
  line L10 (-15, -57) -> (-15, -52)
  line L11 (-15, -52) -> (-18, -52)
  line L12 (-18, -52) -> (-18, -20.0531)
  line L13 (-18, -20.0531) -> (-15, -20.0531)
  circle A0 centre (-69.9244, -71.5419) radius 4.9244
  circle A1 centre (-69.7753, -0.5084) radius 4.7753
  constraint tangent L8 A0
  constraint tangent L2 A1
sketch "Sketch56" plane through (0, 0, 20) normal (0, 0, 1) x (-1, 0, 0)
  line L0 (0, -47.5) -> (0, -57.5)
  line L1 (0, -57.5) -> (1.5, -57.5)
  line L2 (1.5, -57.5) -> (1.5, -14.5)
  line L3 (1.5, -14.5) -> (0, -14.5)
  line L4 (0, -14.5) -> (0, -24.5)
  line L5 (0, -24.5) -> (-25, -24.5)
  line L6 (-25, -24.5) -> (-25, -47.5)
  line L7 (-25, -47.5) -> (0, -47.5)
  line L8 (-25, -47.5) -> (-70, -70)
  line L9 (-70, -70) -> (-25, -24.5)
  line L10 (-25, -24.5) -> (-70, 0)
  line L11 (-70, 0) -> (-25, -47.5)
  constraint coincident L6.end L7.start
  constraint coincident L5.end L6.start
extrude "Extrude57" add sketch "Sketch55" along normal blind 27 contours A1 | A0 bodies 24
sketch "Sketch57" plane through (0, 0, 5) normal (0, 0, 1) x (-1, 0, 0)
  circle A0 centre (-69.9244, -71.5419) radius 4.9244
  circle A1 centre (-69.9244, -71.5419) radius 1.5
  dimension "d162" = 3
  constraint concentric A0 A1
  measures "d162" diameter of A1
sketch "Sketch58" plane through (0, 0, 5) normal (0, 0, 1) x (-1, 0, 0)
  circle A0 centre (-69.7753, -0.5084) radius 4.7753
  circle A1 centre (-69.7753, -0.5084) radius 1.5
  dimension "d163" = 3
  constraint concentric A0 A1
  measures "d163" diameter of A1
extrude "Extrude58" cut sketch "Sketch57" sketch "Sketch58" against normal blind 55 contours A1 of sketch 2 contours A1 bodies 24
sketch "Sketch59" plane through (0, 0, 5) normal (0, 0, 1) x (-1, 0, 0)
  circle A0 centre (-69.9244, -71.5419) radius 1.5
  circle A1 centre (-69.9244, -71.5419) radius 4.9244
  line L0 (-65, -86) -> (-83, -86)
  line L1 (-83, -86) -> (-96.5, -72)
  line L2 (-96.5, -72) -> (-96.5, 0)
  line L3 (-96.5, 0) -> (-83, 14)
  line L4 (-83, 14) -> (-65, 14)
  line L5 (-65, 14) -> (-65, -15)
  line L6 (-65, -15) -> (-26, -15)
  line L7 (-26, -15) -> (-26, -57)
  line L8 (-26, -57) -> (-65, -57)
  line L9 (-65, -57) -> (-65, -86)
  line L10 (-75, -60) -> (-96.5, -60)
  line L11 (-75, -60) -> (-75, -12)
  line L12 (-75, -12) -> (-96.5, -12)
  constraint horizontal L0
  constraint perpendicular L0 L2
  constraint perpendicular L2 L4
  constraint perpendicular L4 L5
  constraint perpendicular L5 L6
  constraint perpendicular L4 L7
  constraint perpendicular L7 L8
  constraint perpendicular L4 L9
  constraint coincident L2 L10.end
  constraint perpendicular L2 L10
  constraint perpendicular L10 L11
  constraint coincident L2 L12.end
  constraint perpendicular L2 L12
extrude "Extrude59" add sketch "Sketch59" along normal blind 1.5 separate body contours A1 | L0 L1 L2 L3 L4 L5 L6 L7 L8 L9 L10 L11 L12 makes body 25
extrude "Extrude60" cut sketch "Sketch58" along normal blind 6 contours A1 bodies 25
move_body "Move26" bodies 23 to x (1, 0, 0) y (0, 1, 0) z (0, 0, 1) at (20, 0, 0)
sketch "Sketch60" plane through (0, 0, 6.5) normal (0, 0, 1) x (-1, 0, 0)
  circle A0 centre (-69.7753, -0.5084) radius 1.5
  circle A1 centre (-69.9244, -71.5419) radius 1.5
  line L0 (-75, -60) -> (-96.5, -60)
  line L1 (-96.5, -60) -> (-96.5, -72)
  line L2 (-96.5, -72) -> (-83, -86)
  line L3 (-83, -86) -> (-65, -86)
  line L4 (-65, -86) -> (-65, -57)
  line L5 (-65, -57) -> (-26, -57)
  line L6 (-26, -57) -> (-26, -15)
  line L7 (-26, -15) -> (-65, -15)
  line L8 (-65, -15) -> (-65, 14)
  line L9 (-65, 14) -> (-83, 14)
  line L10 (-83, 14) -> (-96.5, 0)
  line L11 (-96.5, 0) -> (-96.5, -12)
  line L12 (-96.5, -12) -> (-75, -12)
  line L13 (-75, -12) -> (-75, -60)
  line L14 (-65, -84) -> (-83, -84)
  line L15 (-83, -84) -> (-95, -72)
  line L16 (-95, -72) -> (-95, -60)
  line L17 (-65, -84) -> (-65, -86)
  line L18 (-83, -86) -> (-96.5, -72)
  line L19 (-96.5, -60) -> (-95, -60)
  constraint coincident L4 L14.start
  constraint perpendicular L4 L14
  constraint coincident L0 L16.end
  constraint perpendicular L0 L16
  constraint coincident L3.end L4.start
  constraint coincident L2.end L3.start
  constraint coincident L1.end L2.start
  constraint coincident L0.end L1.start
sketch "Sketch61" plane through (0, 0, 6.5) normal (0, 0, 1) x (-1, 0, 0)
  line L0 (-65, 12) -> (-83, 12)
  line L1 (-83, 12) -> (-95, 0)
  line L2 (-95, 0) -> (-95, -12)
  line L3 (-95, -12) -> (-96, -12)
  line L4 (-96, -12) -> (-96.5, -12)
  line L5 (-96.5, -12) -> (-96.5, 0)
  line L6 (-96.5, 0) -> (-83, 14)
  line L7 (-83, 14) -> (-65, 14)
  line L8 (-65, 14) -> (-65, 12)
  constraint horizontal L0
  constraint perpendicular L0 L2
  constraint perpendicular L2 L3
  constraint perpendicular L2 L4
  constraint perpendicular L4 L5
  constraint perpendicular L5 L7
  constraint perpendicular L0 L8
extrude "Extrude61" add sketch "Sketch60" sketch "Sketch61" along normal blind 14 contours L0 L1 L2 L3 L4 L14 L15 L16 L17 L18 L19 of sketch 2 bodies 25
sketch "Sketch62" plane through (0, 0, 6.5) normal (0, 0, 1) x (-1, 0, 0)
  line L0 (-95, 0) -> (-95, -12)
  line L1 (-95, -12) -> (-75, -12)
  line L2 (-75, -12) -> (-75, -60)
  line L3 (-75, -60) -> (-95, -60)
  line L4 (-95, -60) -> (-95, -72)
  line L5 (-95, -72) -> (-83, -84)
  line L6 (-83, -84) -> (-65, -84)
  line L7 (-65, -84) -> (-65, -57)
  line L8 (-65, -57) -> (-26, -57)
  line L9 (-26, -57) -> (-26, -15)
  line L10 (-26, -15) -> (-65, -15)
  line L11 (-65, -15) -> (-65, 12)
  line L12 (-65, 12) -> (-83, 12)
  line L13 (-83, 12) -> (-95, 0)
  circle A0 centre (-69.9244, -71.5419) radius 1.5
  circle A1 centre (-69.7753, -0.5084) radius 1.5
  line L14 (-95, -62) -> (-75, -62)
  line L15 (-75, -62) -> (-75, -60)
  line L16 (-95, -60) -> (-95, -62)
  line L17 (-95, -60) -> (-75, -60)
  line L18 (-95, -62) -> (-95, -60)
  line L19 (-95, -10) -> (-75, -10)
  line L20 (-75, -10) -> (-75, -12)
  constraint coincident L4 L14.start
  constraint perpendicular L4 L14
  constraint coincident L2.end L3.start
  constraint perpendicular L3 L15
  constraint coincident L3.end L4.start
  constraint perpendicular L14 L16
  constraint perpendicular L17 L18
  constraint coincident L0 L19.start
  constraint perpendicular L0 L19
  constraint coincident L1.end L2.start
  constraint perpendicular L1 L20
extrude "Extrude62" add sketch "Sketch62" along normal blind 14 contours L0 L1 L19 L20 | L3 L4 L14 L15 L16 L17 L18 bodies 25